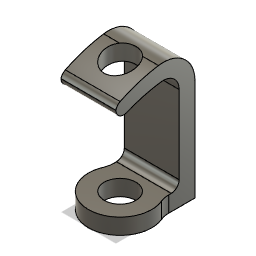
WireHolder v3 (Autodesk Fusion 360 design; units mm, degrees)
Autodesk Fusion 360 part; units mm, degrees
sketch "Sketch1" plane through (0, 0, 0) normal (0, 1, 0) x (1, 0, 0)
  circle A0 centre (0, 0) radius 2
  circle A1 centre (0, 0) radius 4
  line L0 (0, 0) -> (0, 2)
  line L1 (0, 2) -> (3.4641, 2)
  line L2 (0, 2) -> (-3.4641, 2)
  line L3 (3.4641, 2) -> (3.4641, 6)
  line L4 (3.4641, 6) -> (-3.4641, 6)
  line L5 (-3.4641, 6) -> (-3.4641, 2)
  line L6 (-3.4641, 2) -> (3.4641, 2)
  line L7 (3.4641, 2) -> (3.4641, 6)
  dimension "d1" = 4
  dimension "d2" = 8
  dimension "d5" = 4
  constraint coincident A0.centre A1.centre
  constraint concentric A0 A1
  constraint coincident A0 L0.end
  constraint vertical L0
  constraint coincident A1 L1.end
  constraint tangent A0 L1
  constraint coincident A1 L2.end
  constraint tangent A0 L2
  constraint perpendicular L1 L3
  constraint horizontal L4
  constraint vertical L5
  constraint horizontal L6
  constraint vertical L7
  measures "d1" diameter of A0
  measures "d2" diameter of A1
  measures "d5" distance of L1.end L3.end
extrude "Extrude1" add sketch "Sketch1" along normal blind 2
sketch "Sketch2" plane through (0, 2, 0) normal (0, 1, 0) x (-1, 0, 0)
  circle A0 centre (0, 0) radius 2
  line L0 (-3.4641, -2) -> (-3.4641, -6)
  line L1 (-3.4641, -6) -> (3.4641, -6)
  line L2 (3.4641, -6) -> (3.4641, -2)
  arc A1 (3.4641, -2) -> (-3.4641, -2) centre (0, 0) ccw
  line L3 (-3.4641, -6) -> (3.4641, -6)
  line L4 (3.4641, -6) -> (3.4641, -4)
  line L5 (3.4641, -4) -> (-3.4641, -4)
  line L6 (-3.4641, -4) -> (-3.4641, -6)
  dimension "d6" = 2
  constraint horizontal L3
  constraint vertical L4
  constraint horizontal L5
  constraint vertical L6
  constraint coincident L0.end L1.start
  measures "d6" distance of L0.end L5.end
extrude "Extrude2" add sketch "Sketch2" along normal blind 15 contours L0 L1 L2 L3 L4 L5 L6
sketch "Sketch3" plane through (3.4641, 0, 0) normal (1, 0, 0) x (0, 0, -1)
  line L0 (2, 0) -> (6, 0)
  line L1 (6, 0) -> (6, 17)
  line L2 (6, 17) -> (4, 17)
  line L3 (4, 17) -> (4, 2)
  line L4 (4, 2) -> (2, 2)
  line L5 (2, 2) -> (2, 0)
  line L6 (4, 17) -> (4, 15)
  line L7 (4, 15) -> (-4, 15)
  line L8 (-4, 15) -> (-4, 13)
  arc A0 (4, 15) -> (-4, 13) centre (4, -2) ccw
  arc A1 (4, 17) -> (-4, 15) centre (4, 0) ccw
  dimension "d9" = 2
  dimension "d10" = 8
  dimension "d11" = 2
  constraint coincident L2.end L3.start
  constraint perpendicular L2 L6
  constraint perpendicular L6 L7
  constraint perpendicular L7 L8
  constraint tangent L7 A0
  constraint tangent L2 A1
  measures "d9" distance of L2.end L6.end
  measures "d10" distance of L6.end L7.end
  measures "d11" distance of L7.end L8.end
extrude "Extrude3" add sketch "Sketch3" against normal blind 6.928 contours L3 L6 L7 A1 | L7 L8 A0
extrude "Extrude4" cut sketch "Sketch1" along normal blind 21 contours A0
fillet "Fillet1" radius 2 1 edges at (0.0001, 15, -4)
fillet "Fillet2" radius 4 1 edges at (0, 17, -6)
fillet "Fillet3" radius 1 2 edges at (0.0001, 13, 4) (0.0001, 15, 4)
fillet "Fillet4" radius 1 1 edges at (0, 2, -4)
fillet "Fillet5" radius 3 2 edges at (-3.4641, 1, -2) (3.4641, 1, -2)
